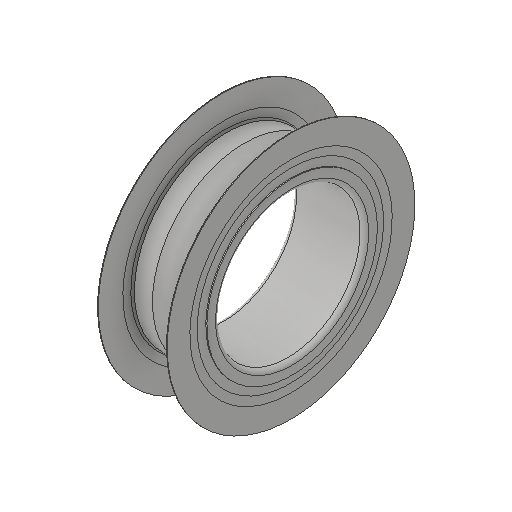
# Autodesk Inventor part: SKF_W 61800 R-2RS1_PART1
Saved by Autodesk Inventor 2022 (Build 260153000, 153)
## iProperties
Category: PARTsolutions
Company: SKF
Created: 2022-07-26
Part Number: SKF_W 61800 R-2RS1_PART1
Material: Generic
Catalog Web Link: www.cadenas.de
Description: -Deep groove ball bearings
Vendor: SKF
Document SubType Name: Modeling
Designer: psAdmin
Manufacturer: SKF
Mass: 6 g
Surface Area: 9.25575 cm^2
Volume: 0.24486 cm^3
Density: 1 g/cm^3
Appearance: PSOLRGB-175-175-175
PSOL_IDENT_0: {$CADENAS_DATA/23d-libs/skf/bearings_units_and_housings/ball_bearings/deep_groove_ball_bearings/bb1_
PSOL_IDENT_1: 001_101.prj},215 {VTYP=3D},{NB=SKF_W 61800 R-2RS1_PART1},{LINA=SKF_W 61800 R-2RS1_PART1},{NN=BB1_001
PSOL_IDENT_2: _101_PART1},{NOPRJ=TRUE},{DATE=08.07.2022 10:24:27},{GEOMDATE=04.07.2022 10:54:51},{VERSION=},{LINEI
PSOL_IDENT_3: D=22520},{WBVAR=},{WBNUMERIC=}  {NB=SKF_W 61800 R-2RS1_PART1},{LINA=SKF_W 61800 R-2RS1_PART1},{KT=DU
PSOL_IDENT_4: MMY},{DESIGNATION=W 61800 R-2RS1},{R12=0.30},{DD=10.000},{D=19.000},{B=5.000},{C=},{CX=},{CXX=1},{CA=
PSOL_IDENT_5: 1.000},{XXVARIANT=Flanged outer ring},{XXDESIGN=Single row stainless steel},{XXSEALING=Contact seal
PSOL_IDENT_6: on both sides},{DESIGN=dgbbwr2zs},{DESIGNIR=dgbbwr2zs},{VARIANT=Flanged outer ring},{DD1=12.74},{DD2=
PSOL_IDENT_7: 11.8},{DD2X=},{DD2A=11.80},{D1=16.26},{D1X=0.00},{D2=17.15},{D2A=17.15},{D3=21},{D3X=},{D3A=21.000},
PSOL_IDENT_8: {D4=},{HH=0.000},{BB=0.000},{BBX=},{BBA=0.000},{FF=},{R0MAX=0.000},{R0=0.000},{PITCH=14.50},{DW=2.38
PSOL_IDENT_9: 1},{DDAMIN=11.500},{DDAMAX=11.500},{DDBMIN=0.000},{DDBMAX=0.000},{DBMIN=0.000},{DAMAX=0.000},{BBAMIN=
PSOL_IDENT_10: 0.000},{CAMAX=0.000},{RAMAX=0.300},{LOAD1=1.480},{LOAD2=0.830},{LOAD3=0.036},{SPEED1=0},{SPEED2=2200
PSOL_IDENT_11: 0},{KR=0.020},{F0=14.800},{Z=10},{II=1},{MASS=0.006},{BEARING=W 61800 R-2RS1},{RING=},{HELP=1.370},{
PSOL_IDENT_12: HELP2=0.925},{DD1ALG=6.370},{YALG=6.370},{PITCH1=14.500},{DW1=2.381},{YALG1=8.130},{HALG1=1.370},{SH=
PSOL_IDENT_13: 5.900},{CU=0.524},{HALG=1.37},{B1=-2.82145},{SHIELDHELP=2},{D4A=0.000},{FFA=0.000},{RS1=},{HELP3=0}
NB: SKF_W 61800 R-2RS1_PART1
NT: Deep groove ball bearings
NBSYN: SKF_$DESIGNATION._PART1
LINA: SKF_W 61800 R-2RS1_PART1
CATALOG: SKF
DESIGNATION: W 61800 R-2RS1
R12: 0.3
DD: 10
D: 19
B: 5
XXVARIANT: Flanged outer ring
XXDESIGN: Single row stainless steel
XXSEALING: Contact seal on both sides
DD2: 11.8
D2: 17.15
LOAD1: 1.48
LOAD2: 0.83
LOAD3: 0.036
SPEED1: 0
SPEED2: 22000
BEARING: W 61800 R-2RS1
SUPPLIER: SKF
ARTICLENO: SKF_W 61800 R-2RS1_PART1
BOMINFO: SKF_W 61800 R-2RS1_PART1
CREATOR: CADENAS GmbH
Title: SKF_W 61800 R-2RS1_PART1
Author: Cadenas PARTsolutions
Comments: Deep groove ball bearings
Autodesk Inventor part; units mm, degrees
ref_plane "YZ Plane" through (0, 0, 0) normal (1, 0, 0) x (0, 1, 0)
ref_plane "XZ Plane" through (0, 0, 0) normal (0, 1, 0) x (-1, 0, 0)
ref_plane "XY Plane" through (0, 0, 0) normal (0, 0, 1) x (1, 0, 0)
sketch "Sketch_40" plane through (0, 0, 0) normal (0, 0, 1) x (1, 0, 0)
  line L0 (2.5, 0) -> (-2.5, 0)
  line L1 (0, 6.295) -> (0, 5.3)
  arc A0 (0, 5.3) -> (0.3, 5) centre (0.3, 5.3) ccw
  line L2 (0.3, 5) -> (4.7, 5)
  arc A1 (4.7, 5) -> (5, 5.3) centre (4.7, 5.3) ccw
  line L3 (5, 5.3) -> (5, 6.295)
  arc A2 (5, 6.295) -> (4.925, 6.37) centre (4.925, 6.295) ccw
  line L4 (4.925, 6.37) -> (3.3018, 6.37)
  arc A3 (1.6982, 6.37) -> (3.3018, 6.37) centre (2.5, 7.25) ccw
  line L5 (1.6982, 6.37) -> (0.075, 6.37)
  arc A4 (0.075, 6.37) -> (0, 6.295) centre (0.075, 6.295) ccw
  constraints: 12 end point, 10 point on circle, 5 centre point
revolve "Revolution1" add sketch "Sketch_40" angle 360 about axis through (2.5, 0, 0) along (1, 0, 0)
sketch "Sketch_42" plane through (0, 0, 0) normal (0, 0, 1) x (1, 0, 0)
  line L0 (2.5, 0) -> (-2.5, 0)
  line L1 (0, 13.15) -> (0, 5.9)
  line L2 (0, 5.9) -> (0.15, 5.9)
  arc A0 (0.15, 5.9) -> (0.45, 6.2) centre (0.15, 6.2) ccw
  line L3 (0.45, 6.2) -> (0.45, 12.85)
  line L4 (0.45, 12.85) -> (4.55, 12.85)
  line L5 (4.55, 12.85) -> (4.55, 6.2)
  arc A1 (4.55, 6.2) -> (4.85, 5.9) centre (4.85, 6.2) ccw
  line L6 (4.85, 5.9) -> (5, 5.9)
  line L7 (5, 5.9) -> (5, 13.15)
  line L8 (5, 13.15) -> (0, 13.15)
  constraints: 18 end point, 4 point on circle, 2 centre point
revolve "Revolution2" cut sketch "Sketch_42" angle 360 about axis through (2.5, 0, 0) along (1, 0, 0)
sketch "Sketch_44" plane through (0, 0, 0) normal (0, 0, 1) x (1, 0, 0)
  line L0 (5, 0) -> (-5, 0)
  line L1 (4.745, 6.4513) -> (4.835, 5.9)
  line L2 (4.835, 5.9) -> (4.925, 5.9)
  line L3 (4.925, 5.9) -> (4.88, 6.4513)
  line L4 (4.88, 6.4513) -> (4.925, 7.0025)
  line L5 (4.925, 7.0025) -> (4.925, 8.575)
  line L6 (4.925, 8.575) -> (4.8734, 8.575)
  line L7 (4.8734, 8.575) -> (4.745, 7.0025)
  line L8 (4.745, 7.0025) -> (4.745, 6.4513)
  constraints: 18 end point
revolve "Revolution3" add sketch "Sketch_44" angle 360 about axis through (5, 0, 0) along (1, 0, 0)
sketch "Sketch_49" plane through (0, 0, 0) normal (0, 0, 1) x (1, 0, 0)
  line L0 (5, 0) -> (-5, 0)
  line L1 (0.105, 5.9) -> (0.195, 5.9)
  line L2 (0.195, 5.9) -> (0.285, 6.4513)
  line L3 (0.285, 6.4513) -> (0.285, 7.0025)
  line L4 (0.285, 7.0025) -> (0.1566, 8.575)
  line L5 (0.1566, 8.575) -> (0.105, 8.575)
  line L6 (0.105, 8.575) -> (0.105, 7.0025)
  line L7 (0.105, 7.0025) -> (0.15, 6.4513)
  line L8 (0.15, 6.4513) -> (0.105, 5.9)
  constraints: 18 end point
revolve "Revolution4" add sketch "Sketch_49" angle 360 about axis through (5, 0, 0) along (1, 0, 0)
body "Solid1"
